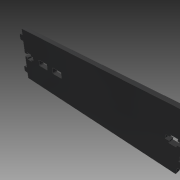
# Autodesk Inventor part: front_panel_2004_front
Saved by Autodesk Inventor 2014 (Build 180170000, 170)
## iProperties
Created: 2014-01-11
Part Number: front_panel_2004_front
Material: Generic
Document SubType Name: Modeling
Designer: buben
Density: 1 g/cm^3
Appearance: Anodized - Dark Gray
Author: buben
Autodesk Inventor part; units mm, degrees
ref_plane "YZ Plane" through (0, 0, 0) normal (1, 0, 0) x (0, 1, 0)
ref_plane "XZ Plane" through (0, 0, 0) normal (0, 1, 0) x (-1, 0, 0)
ref_plane "XY Plane" through (0, 0, 0) normal (0, 0, 1) x (1, 0, 0)
sketch "Sketch1" plane through (0, 0, 0) normal (0, 1, 0) x (-1, 0, 0)
  line L0 (0, 0) -> (220, 0)
  line L1 (220, 0) -> (220, 68.618)
  line L2 (220, 68.618) -> (0, 68.618)
  line L3 (0, 68.618) -> (0, 0)
  dimension "d0" = 68.618
  dimension "d1" = 220
  constraints: 8 end point, 2 parallel, 1 horizontal, 1 perpendicular
  measures "d0" distance of L2.end L0.start
  measures "d1" distance of L1.end L2.end
extrude "Extrusion1" add sketch "Sketch1" along normal blind 6
sketch "Sketch2" plane through (0, 6, 0) normal (0, 1, 0) x (1, 0, 0)
  line L0 (-220, 0) -> (-220, -68.618) projected
  line L1 (0, -68.618) -> (0, 0) projected
  line L2 (-220, -8) -> (-224, -8)
  line L3 (-226, -10) -> (-226, -14)
  line L4 (-224, -16) -> (-220, -16)
  line L5 (-220, -16) -> (-220, -8)
  line L6 (-220, -52.618) -> (-224, -52.618)
  line L7 (-226, -54.618) -> (-226, -58.618)
  line L8 (-224, -60.618) -> (-220, -60.618)
  line L9 (-220, -60.618) -> (-220, -52.618)
  line L10 (0, -8) -> (4, -8)
  line L11 (6, -10) -> (6, -14)
  line L12 (4, -16) -> (0, -16)
  line L13 (0, -16) -> (0, -8)
  line L14 (0, -52.618) -> (4, -52.618)
  line L15 (6, -54.618) -> (6, -58.618)
  line L16 (4, -60.618) -> (0, -60.618)
  line L17 (0, -60.618) -> (0, -52.618)
  arc A0 (-224, -8) -> (-226, -10) centre (-224, -10) ccw
  arc A1 (-226, -14) -> (-224, -16) centre (-224, -14) ccw
  arc A2 (-224, -52.618) -> (-226, -54.618) centre (-224, -54.618) ccw
  arc A3 (-226, -58.618) -> (-224, -60.618) centre (-224, -58.618) ccw
  arc A4 (4, -60.618) -> (6, -58.618) centre (4, -58.618) ccw
  arc A5 (6, -54.618) -> (4, -52.618) centre (4, -54.618) ccw
  arc A6 (4, -16) -> (6, -14) centre (4, -14) ccw
  arc A7 (6, -10) -> (4, -8) centre (4, -10) ccw
  line L18 (-222, -16) -> (-222, -52.618) construction
  line L19 (0, 0) -> (-220, 0) projected
  point P0 (-222, -34.309)
  point P1 (-220, -34.309)
  dimension "d4" = 2
  dimension "d5" = 8
  dimension "d6" = 8
  dimension "d7" = 6
  dimension "d8" = 6
  dimension "d41" = 8
  constraints: 34 end point, 16 point on circle, 16 tangent, 8 centre point, 8 parallel, 7 equal radius, 6 collinear, 4 horizontal, 4 midpoint, 4 perpendicular, 4 point on line, 1 horizontal alignment
  measures "d4" radius of A0
  measures "d5" distance between parallel lines of L4 L2
  measures "d6" distance between parallel lines of L8 L6
  measures "d7" distance between parallel lines of L0 L3
  measures "d8" distance between parallel lines of L1 L11
  measures "d41" distance between parallel lines of L19 L2
extrude "Extrusion2" add sketch "Sketch2" against normal blind 6
sketch "Sketch3" plane through (0, 6, 0) normal (0, 1, 0) x (1, 0, 0)
  line L0 (0, 0) -> (-220, 0) projected
  line L1 (-220, -16) -> (-220, -52.618) projected
  line L2 (-220, -68.618) -> (0, -68.618) projected
  line L3 (-203.7, -32.059) -> (-203.7, -36.559)
  line L4 (-220, -36.559) -> (-220, -32.059)
  line L5 (-215, -29.559) -> (-207.7, -29.559)
  line L6 (-207.7, -39.059) -> (-215, -39.059)
  line L7 (-220, -32.059) -> (-215, -32.059)
  line L8 (-207.7, -32.059) -> (-203.7, -32.059)
  line L9 (-203.7, -36.559) -> (-207.7, -36.559)
  line L10 (-215, -36.559) -> (-220, -36.559)
  line L11 (-207.7, -29.559) -> (-207.7, -32.059)
  line L12 (-207.7, -36.559) -> (-207.7, -39.059)
  line L13 (-215, -39.059) -> (-215, -36.559)
  line L14 (-215, -32.059) -> (-215, -29.559)
  line L15 (-110, 0) -> (-110, -68.618) construction
  line L16 (-16.3, -32.059) -> (-16.3, -36.559)
  line L17 (0, -36.559) -> (0, -32.059)
  line L18 (-5, -29.559) -> (-12.3, -29.559)
  line L19 (-12.3, -39.059) -> (-5, -39.059)
  line L20 (0, -32.059) -> (-5, -32.059)
  line L21 (-12.3, -32.059) -> (-16.3, -32.059)
  line L22 (-16.3, -36.559) -> (-12.3, -36.559)
  line L23 (-5, -36.559) -> (0, -36.559)
  line L24 (-12.3, -29.559) -> (-12.3, -32.059)
  line L25 (-12.3, -36.559) -> (-12.3, -39.059)
  line L26 (-5, -39.059) -> (-5, -36.559)
  line L27 (-5, -32.059) -> (-5, -29.559)
  point P0 (-203.7, -34.309)
  point P1 (-220, -34.309)
  point P2 (-16.3, -34.309)
  point P3 (0, -34.309)
  dimension "d12" = 4.5
  dimension "d13" = 2.5
  dimension "d14" = 2.5
  dimension "d15" = 5
  dimension "d16" = 4
  dimension "d17" = 7.3
  constraints: 50 end point, 14 symmetric about line, 10 parallel, 5 collinear, 4 midpoint, 4 perpendicular, 3 horizontal, 1 horizontal alignment
  measures "d12" distance of L3.start L3.end
  measures "d13" distance of L5.end L8.start
  measures "d14" distance of L9.end L6.start
  measures "d15" distance of L10.start L4.start
  measures "d16" distance of L3.end L9.end
  measures "d17" distance of L6.start L6.end
extrude "Extrusion3" cut sketch "Sketch3" against normal blind 6
sketch "Sketch4" plane through (0, 0, 0) normal (0, -1, 0) x (1, 0, 0)
  line L0 (-203.7, 36.559) -> (-203.7, 32.059) projected
  line L1 (-190.7, 38.309) -> (-177.7, 38.309)
  line L2 (-176.7, 37.309) -> (-176.7, 31.309)
  line L3 (-177.7, 30.309) -> (-190.7, 30.309)
  line L4 (-191.7, 31.309) -> (-191.7, 37.309)
  line L5 (-165.7, 38.309) -> (-152.7, 38.309)
  line L6 (-151.7, 37.309) -> (-151.7, 31.309)
  line L7 (-152.7, 30.309) -> (-165.7, 30.309)
  line L8 (-166.7, 31.309) -> (-166.7, 37.309)
  arc A0 (-190.7, 38.309) -> (-191.7, 37.309) centre (-190.7, 37.309) ccw
  arc A1 (-176.7, 37.309) -> (-177.7, 38.309) centre (-177.7, 37.309) ccw
  arc A2 (-177.7, 30.309) -> (-176.7, 31.309) centre (-177.7, 31.309) ccw
  arc A3 (-191.7, 31.309) -> (-190.7, 30.309) centre (-190.7, 31.309) ccw
  arc A4 (-165.7, 38.309) -> (-166.7, 37.309) centre (-165.7, 37.309) ccw
  arc A5 (-151.7, 37.309) -> (-152.7, 38.309) centre (-152.7, 37.309) ccw
  arc A6 (-152.7, 30.309) -> (-151.7, 31.309) centre (-152.7, 31.309) ccw
  arc A7 (-166.7, 31.309) -> (-165.7, 30.309) centre (-165.7, 31.309) ccw
  point P0 (-203.7, 34.309)
  point P1 (-191.7, 34.309)
  dimension "d20" = 1
  dimension "d21" = 15
  dimension "d22" = 15
  dimension "d23" = 8
  dimension "d24" = 10
  dimension "d25" = 12
  constraints: 16 end point, 16 point on circle, 16 tangent, 8 centre point, 7 equal radius, 4 parallel, 2 collinear, 2 horizontal, 2 midpoint, 2 perpendicular, 1 horizontal alignment
  measures "d20" radius of A0
  measures "d21" distance between parallel lines of L2 L4
  measures "d22" distance between parallel lines of L6 L8
  measures "d23" distance between parallel lines of L3 L1
  measures "d24" distance between parallel lines of L8 L2
  measures "d25" distance between parallel lines of L0 L4
extrude "Extrusion4" cut sketch "Sketch4" against normal through all
sketch "Sketch6" plane through (0, 6, 0) normal (0, 1, 0) x (1, 0, 0)
  line L0 (-220, -68.618) -> (0, -68.618) projected
  line L1 (0, -68.618) -> (0, -60.618) projected
  line L2 (-50, -52.618) -> (-10, -52.618) construction
  line L3 (-10, -52.618) -> (-10, -62.618) construction
  line L4 (-10, -62.618) -> (-50, -62.618) construction
  line L5 (-50, -62.618) -> (-50, -52.618) construction
  spline S0 degree 2 poles (-43.1283, -54.9198) (-43.1283, -55.8013) (-43.8661, -56.3008) knots 0 0 0 1 1 1
  spline S1 degree 2 poles (-43.8661, -56.3008) (-44.16, -56.4967) (-44.5518, -56.4967) knots 0 0 0 1 1 1
  line L6 (-44.5518, -56.4967) -> (-45.9035, -56.4967)
  spline S2 degree 2 poles (-45.9035, -56.4967) (-46.07, -56.4967) (-46.07, -56.3694) knots 0 0 0 1 1 1
  spline S3 degree 2 poles (-46.07, -56.3694) (-46.07, -56.2453) (-45.9035, -56.2453) knots 0 0 0 1 1 1
  line L7 (-45.9035, -56.2453) -> (-45.6912, -56.2453)
  line L8 (-45.6912, -56.2453) -> (-45.6912, -53.2481)
  line L9 (-45.6912, -53.2481) -> (-45.9035, -53.2481)
  spline S4 degree 2 poles (-45.9035, -53.2481) (-46.07, -53.2481) (-46.07, -53.1208) knots 0 0 0 1 1 1
  spline S5 degree 2 poles (-46.07, -53.1208) (-46.07, -52.9967) (-45.9035, -52.9967) knots 0 0 0 1 1 1
  line L10 (-45.9035, -52.9967) -> (-44.5518, -52.9967)
  spline S6 degree 2 poles (-44.5518, -52.9967) (-43.9282, -52.9967) (-43.5723, -53.4277) knots 0 0 0 1 1 1
  spline S7 degree 2 poles (-43.5723, -53.4277) (-43.1283, -53.9664) (-43.1283, -54.5737) knots 0 0 0 1 1 1
  line L11 (-43.1283, -54.5737) -> (-43.1283, -54.9198)
  line L12 (-43.3797, -54.9753) -> (-43.3797, -54.5182)
  spline S8 degree 2 poles (-43.3797, -54.5182) (-43.3797, -54.2864) (-43.4548, -54.1035) knots 0 0 0 1 1 1
  spline S9 degree 2 poles (-43.4548, -54.1035) (-43.5625, -53.8358) (-43.7584, -53.5975) knots 0 0 0 1 1 1
  spline S10 degree 2 poles (-43.7584, -53.5975) (-44.0457, -53.2481) (-44.5289, -53.2481) knots 0 0 0 1 1 1
  line L13 (-44.5289, -53.2481) -> (-45.4398, -53.2481)
  line L14 (-45.4398, -53.2481) -> (-45.4398, -56.2453)
  line L15 (-45.4398, -56.2453) -> (-44.5289, -56.2453)
  spline S11 degree 2 poles (-44.5289, -56.2453) (-44.2155, -56.2453) (-43.9314, -56.0364) knots 0 0 0 1 1 1
  spline S12 degree 2 poles (-43.9314, -56.0364) (-43.6604, -55.8405) (-43.5168, -55.5434) knots 0 0 0 1 1 1
  spline S13 degree 2 poles (-43.5168, -55.5434) (-43.3797, -55.2561) (-43.3797, -54.9753) knots 0 0 0 1 1 1
  spline S14 degree 2 poles (-39.6642, -56.0854) (-39.6642, -56.1343) (-39.7132, -56.1866) knots 0 0 0 1 1 1
  spline S15 degree 2 poles (-39.7132, -56.1866) (-39.896, -56.3727) (-40.3041, -56.4935) knots 0 0 0 1 1 1
  spline S16 degree 2 poles (-40.3041, -56.4935) (-40.66, -56.5947) (-40.9734, -56.5947) knots 0 0 0 1 1 1
  spline S17 degree 2 poles (-40.9734, -56.5947) (-41.6035, -56.5947) (-42.0378, -56.1866) knots 0 0 0 1 1 1
  spline S18 degree 2 poles (-42.0378, -56.1866) (-42.4851, -55.7719) (-42.4851, -55.1483) knots 0 0 0 1 1 1
  spline S19 degree 2 poles (-42.4851, -55.1483) (-42.4851, -54.5737) (-42.0639, -54.1884) knots 0 0 0 1 1 1
  spline S20 degree 2 poles (-42.0639, -54.1884) (-41.6525, -53.8162) (-41.0779, -53.8162) knots 0 0 0 1 1 1
  spline S21 degree 2 poles (-41.0779, -53.8162) (-40.4445, -53.8162) (-39.6642, -54.6292) (-39.6707, -55.2626) knots 0 0 0 1 2 2 2
  line L16 (-39.6707, -55.2626) -> (-42.2304, -55.2626)
  spline S22 degree 2 poles (-42.2304, -55.2626) (-42.1651, -55.7589) (-41.4762, -56.3433) (-40.9734, -56.3433) knots 0 0 0 1 2 2 2
  spline S23 degree 2 poles (-40.9734, -56.3433) (-40.3139, -56.3433) (-39.8829, -56.007) knots 0 0 0 1 1 1
  spline S24 degree 2 poles (-39.8829, -56.007) (-39.8242, -55.9613) (-39.785, -55.9613) knots 0 0 0 1 1 1
  spline S25 degree 2 poles (-39.785, -55.9613) (-39.6642, -55.9613) (-39.6642, -56.0854) knots 0 0 0 1 1 1
  spline S26 degree 2 poles (-39.9254, -55.0079) (-40.0005, -54.5835) (-40.6437, -54.0709) (-41.0746, -54.0709) knots 0 0 0 1 2 2 2
  spline S27 degree 2 poles (-41.0746, -54.0709) (-41.5121, -54.0709) (-42.1488, -54.5802) (-42.2271, -55.0079) knots 0 0 0 1 2 2 2
  line L17 (-42.2271, -55.0079) -> (-39.9254, -55.0079)
  spline S28 degree 2 poles (-36.1348, -55.7752) (-36.1348, -56.1931) (-36.5527, -56.4151) knots 0 0 0 1 1 1
  spline S29 degree 2 poles (-36.5527, -56.4151) (-36.8923, -56.5947) (-37.3461, -56.5947) knots 0 0 0 1 1 1
  spline S30 degree 2 poles (-37.3461, -56.5947) (-37.9403, -56.5947) (-38.319, -56.2943) knots 0 0 0 1 1 1
  spline S31 degree 2 poles (-38.319, -56.2943) (-38.319, -56.4412) (-38.3713, -56.4771) knots 0 0 0 1 1 1
  spline S32 degree 2 poles (-38.3713, -56.4771) (-38.4072, -56.4967) (-38.4431, -56.4967) knots 0 0 0 1 1 1
  spline S33 degree 2 poles (-38.4431, -56.4967) (-38.5704, -56.4967) (-38.5704, -56.3302) knots 0 0 0 1 1 1
  line L18 (-38.5704, -56.3302) -> (-38.5704, -55.8111)
  spline S34 degree 2 poles (-38.5704, -55.8111) (-38.5704, -55.6446) (-38.4431, -55.6446) knots 0 0 0 1 1 1
  spline S35 degree 2 poles (-38.4431, -55.6446) (-38.3158, -55.6446) (-38.3158, -55.7817) knots 0 0 0 1 1 1
  spline S36 degree 2 poles (-38.3158, -55.7817) (-38.3158, -56.0821) (-37.9109, -56.2486) knots 0 0 0 1 1 1
  spline S37 degree 2 poles (-37.9109, -56.2486) (-37.6856, -56.3433) (-37.3526, -56.3433) knots 0 0 0 1 1 1
  spline S38 degree 2 poles (-37.3526, -56.3433) (-37.0163, -56.3433) (-36.7486, -56.2257) knots 0 0 0 1 1 1
  spline S39 degree 2 poles (-36.7486, -56.2257) (-36.3862, -56.0723) (-36.3862, -55.7752) knots 0 0 0 1 1 1
  spline S40 degree 2 poles (-36.3862, -55.7752) (-36.3862, -55.3116) (-37.3396, -55.2136) knots 0 0 0 1 1 1
  spline S41 degree 2 poles (-37.3396, -55.2136) (-37.715, -55.1744) (-37.8783, -55.1287) knots 0 0 0 1 1 1
  spline S42 degree 2 poles (-37.8783, -55.1287) (-38.1884, -55.0438) (-38.3288, -54.8545) knots 0 0 0 1 1 1
  spline S43 degree 2 poles (-38.3288, -54.8545) (-38.4431, -54.6978) (-38.4431, -54.5182) knots 0 0 0 1 1 1
  spline S44 degree 2 poles (-38.4431, -54.5182) (-38.4431, -54.1623) (-38.0644, -53.9697) knots 0 0 0 1 1 1
  spline S45 degree 2 poles (-38.0644, -53.9697) (-37.7607, -53.8162) (-37.3689, -53.8162) knots 0 0 0 1 1 1
  spline S46 degree 2 poles (-37.3689, -53.8162) (-36.8498, -53.8162) (-36.5233, -54.0676) knots 0 0 0 1 1 1
  spline S47 degree 2 poles (-36.5233, -54.0676) (-36.5233, -53.9044) (-36.396, -53.9044) knots 0 0 0 1 1 1
  spline S48 degree 2 poles (-36.396, -53.9044) (-36.2687, -53.9044) (-36.2687, -54.0742) knots 0 0 0 1 1 1
  line L19 (-36.2687, -54.0742) -> (-36.2687, -54.5084)
  spline S49 degree 2 poles (-36.2687, -54.5084) (-36.2687, -54.6749) (-36.396, -54.6749) knots 0 0 0 1 1 1
  spline S50 degree 2 poles (-36.396, -54.6749) (-36.5103, -54.6749) (-36.5233, -54.5345) knots 0 0 0 1 1 1
  spline S51 degree 2 poles (-36.5233, -54.5345) (-36.5396, -54.3549) (-36.7094, -54.2374) knots 0 0 0 1 1 1
  spline S52 degree 2 poles (-36.7094, -54.2374) (-36.951, -54.0709) (-37.3559, -54.0709) knots 0 0 0 1 1 1
  spline S53 degree 2 poles (-37.3559, -54.0709) (-37.7803, -54.0709) (-38.0121, -54.2407) knots 0 0 0 1 1 1
  spline S54 degree 2 poles (-38.0121, -54.2407) (-38.1884, -54.3713) (-38.1884, -54.528) knots 0 0 0 1 1 1
  spline S55 degree 2 poles (-38.1884, -54.528) (-38.1884, -54.7076) (-37.9795, -54.8284) knots 0 0 0 1 1 1
  spline S56 degree 2 poles (-37.9795, -54.8284) (-37.8326, -54.91) (-37.4342, -54.9557) knots 0 0 0 1 1 1
  spline S57 degree 2 poles (-37.4342, -54.9557) (-36.9053, -55.0145) (-36.7094, -55.083) knots 0 0 0 1 1 1
  spline S58 degree 2 poles (-36.7094, -55.083) (-36.1348, -55.292) (-36.1348, -55.7752) knots 0 0 0 1 1 1
  spline S59 degree 2 poles (-32.3867, -56.3694) (-32.3867, -56.4967) (-32.5564, -56.4967) knots 0 0 0 1 1 1
  line L20 (-32.5564, -56.4967) -> (-34.7831, -56.4967)
  spline S60 degree 2 poles (-34.7831, -56.4967) (-34.9496, -56.4967) (-34.9496, -56.3694) knots 0 0 0 1 1 1
  spline S61 degree 2 poles (-34.9496, -56.3694) (-34.9496, -56.2453) (-34.7831, -56.2453) knots 0 0 0 1 1 1
  line L21 (-34.7831, -56.2453) -> (-33.7938, -56.2453)
  line L22 (-33.7938, -56.2453) -> (-33.7938, -54.1623)
  line L23 (-33.7938, -54.1623) -> (-34.5285, -54.1623)
  spline S62 degree 2 poles (-34.5285, -54.1623) (-34.6982, -54.1623) (-34.6982, -54.035) knots 0 0 0 1 1 1
  spline S63 degree 2 poles (-34.6982, -54.035) (-34.6982, -53.9076) (-34.5285, -53.9076) knots 0 0 0 1 1 1
  line L24 (-34.5285, -53.9076) -> (-33.5424, -53.9076)
  line L25 (-33.5424, -53.9076) -> (-33.5424, -56.2453)
  line L26 (-33.5424, -56.2453) -> (-32.5564, -56.2453)
  spline S64 degree 2 poles (-32.5564, -56.2453) (-32.3867, -56.2453) (-32.3867, -56.3694) knots 0 0 0 1 1 1
  line L27 (-33.549, -53.2677) -> (-33.9212, -53.2677)
  line L28 (-33.9212, -53.2677) -> (-33.9212, -52.618)
  line L29 (-33.9212, -52.618) -> (-33.549, -52.618)
  line L30 (-33.549, -52.618) -> (-33.549, -53.2677)
  spline S65 degree 2 poles (-28.3969, -54.035) (-28.3969, -54.1623) (-28.5634, -54.1623) knots 0 0 0 1 1 1
  line L31 (-28.5634, -54.1623) -> (-28.903, -54.1623)
  line L32 (-28.903, -54.1623) -> (-28.903, -56.6698)
  spline S66 degree 2 poles (-28.903, -56.6698) (-28.903, -56.9212) (-29.0107, -57.1171) knots 0 0 0 1 1 1
  spline S67 degree 2 poles (-29.0107, -57.1171) (-29.1772, -57.424) (-29.556, -57.5905) knots 0 0 0 1 1 1
  spline S68 degree 2 poles (-29.556, -57.5905) (-29.6931, -57.6493) (-29.9249, -57.6493) knots 0 0 0 1 1 1
  line L33 (-29.9249, -57.6493) -> (-30.6367, -57.6493)
  spline S69 degree 2 poles (-30.6367, -57.6493) (-30.8032, -57.6493) (-30.8032, -57.5219) knots 0 0 0 1 1 1
  spline S70 degree 2 poles (-30.8032, -57.5219) (-30.8032, -57.3946) (-30.6367, -57.3946) knots 0 0 0 1 1 1
  line L34 (-30.6367, -57.3946) -> (-29.9151, -57.3979)
  spline S71 degree 2 poles (-29.9151, -57.3979) (-29.458, -57.4011) (-29.2197, -56.9538) knots 0 0 0 1 1 1
  spline S72 degree 2 poles (-29.2197, -56.9538) (-29.1544, -56.8298) (-29.1544, -56.6339) knots 0 0 0 1 1 1
  line L35 (-29.1544, -56.6339) -> (-29.1544, -55.8797)
  spline S73 degree 2 poles (-29.1544, -55.8797) (-29.5592, -56.4347) (-30.1959, -56.4347) knots 0 0 0 1 1 1
  spline S74 degree 2 poles (-30.1959, -56.4347) (-30.7281, -56.4347) (-31.097, -56.0429) knots 0 0 0 1 1 1
  spline S75 degree 2 poles (-31.097, -56.0429) (-31.4627, -55.6609) (-31.4627, -55.1255) knots 0 0 0 1 1 1
  spline S76 degree 2 poles (-31.4627, -55.1255) (-31.4627, -54.5868) (-30.7281, -53.8162) (-30.1959, -53.8162) knots 0 0 0 1 2 2 2
  spline S77 degree 2 poles (-30.1959, -53.8162) (-29.5592, -53.8162) (-29.1544, -54.368) knots 0 0 0 1 1 1
  line L36 (-29.1544, -54.368) -> (-29.1544, -53.9076)
  line L37 (-29.1544, -53.9076) -> (-28.5634, -53.9076)
  spline S78 degree 2 poles (-28.5634, -53.9076) (-28.3969, -53.9076) (-28.3969, -54.035) knots 0 0 0 1 1 1
  spline S79 degree 2 poles (-29.1544, -55.1255) (-29.1544, -54.688) (-29.7486, -54.0709) (-30.1828, -54.0709) knots 0 0 0 1 2 2 2
  spline S80 degree 2 poles (-30.1828, -54.0709) (-30.6171, -54.0709) (-31.208, -54.6912) (-31.208, -55.1255) knots 0 0 0 1 2 2 2
  spline S81 degree 2 poles (-31.208, -55.1255) (-31.208, -55.5597) (-30.6171, -56.18) (-30.1828, -56.18) knots 0 0 0 1 2 2 2
  spline S82 degree 2 poles (-30.1828, -56.18) (-29.7486, -56.18) (-29.1544, -55.5597) (-29.1544, -55.1255) knots 0 0 0 1 2 2 2
  spline S83 degree 2 poles (-24.8414, -56.3694) (-24.8414, -56.4967) (-25.0079, -56.4967) knots 0 0 0 1 1 1
  line L38 (-25.0079, -56.4967) -> (-25.6805, -56.4967)
  spline S84 degree 2 poles (-25.6805, -56.4967) (-25.8503, -56.4967) (-25.8503, -56.3694) knots 0 0 0 1 1 1
  spline S85 degree 2 poles (-25.8503, -56.3694) (-25.8503, -56.2453) (-25.6805, -56.2453) knots 0 0 0 1 1 1
  line L39 (-25.6805, -56.2453) -> (-25.4715, -56.2453)
  line L40 (-25.4715, -56.2453) -> (-25.4715, -54.7043)
  spline S86 degree 2 poles (-25.4715, -54.7043) (-25.4715, -54.4104) (-25.687, -54.2341) knots 0 0 0 1 1 1
  spline S87 degree 2 poles (-25.687, -54.2341) (-25.8862, -54.0709) (-26.1866, -54.0709) knots 0 0 0 1 1 1
  spline S88 degree 2 poles (-26.1866, -54.0709) (-26.4902, -54.0709) (-26.7285, -54.2472) knots 0 0 0 1 1 1
  spline S89 degree 2 poles (-26.7285, -54.2472) (-26.8657, -54.3484) (-27.1367, -54.6684) knots 0 0 0 1 1 1
  line L41 (-27.1367, -54.6684) -> (-27.1367, -56.2453)
  line L42 (-27.1367, -56.2453) -> (-26.8526, -56.2453)
  spline S90 degree 2 poles (-26.8526, -56.2453) (-26.6861, -56.2453) (-26.6861, -56.3694) knots 0 0 0 1 1 1
  spline S91 degree 2 poles (-26.6861, -56.3694) (-26.6861, -56.4967) (-26.8526, -56.4967) knots 0 0 0 1 1 1
  line L43 (-26.8526, -56.4967) -> (-27.6721, -56.4967)
  spline S92 degree 2 poles (-27.6721, -56.4967) (-27.8386, -56.4967) (-27.8386, -56.3694) knots 0 0 0 1 1 1
  spline S93 degree 2 poles (-27.8386, -56.3694) (-27.8386, -56.2453) (-27.6721, -56.2453) knots 0 0 0 1 1 1
  line L44 (-27.6721, -56.2453) -> (-27.3881, -56.2453)
  line L45 (-27.3881, -56.2453) -> (-27.3881, -54.1623)
  line L46 (-27.3881, -54.1623) -> (-27.6003, -54.1623)
  spline S94 degree 2 poles (-27.6003, -54.1623) (-27.7668, -54.1623) (-27.7668, -54.035) knots 0 0 0 1 1 1
  spline S95 degree 2 poles (-27.7668, -54.035) (-27.7668, -53.9076) (-27.6003, -53.9076) knots 0 0 0 1 1 1
  line L47 (-27.6003, -53.9076) -> (-27.1367, -53.9076)
  line L48 (-27.1367, -53.9076) -> (-27.1367, -54.2864)
  spline S96 degree 2 poles (-27.1367, -54.2864) (-26.673, -53.8162) (-26.1833, -53.8162) knots 0 0 0 1 1 1
  spline S97 degree 2 poles (-26.1833, -53.8162) (-25.6283, -53.8162) (-25.354, -54.2341) knots 0 0 0 1 1 1
  spline S98 degree 2 poles (-25.354, -54.2341) (-25.2201, -54.4431) (-25.2201, -54.6618) knots 0 0 0 1 1 1
  line L49 (-25.2201, -54.6618) -> (-25.2201, -56.2453)
  line L50 (-25.2201, -56.2453) -> (-25.0079, -56.2453)
  spline S99 degree 2 poles (-25.0079, -56.2453) (-24.8414, -56.2453) (-24.8414, -56.3694) knots 0 0 0 1 1 1
  spline S100 degree 2 poles (-17.4855, -55.194) (-17.4855, -55.7621) (-17.8643, -56.1735) knots 0 0 0 1 1 1
  spline S101 degree 2 poles (-17.8643, -56.1735) (-18.2528, -56.5947) (-18.8209, -56.5947) knots 0 0 0 1 1 1
  spline S102 degree 2 poles (-18.8209, -56.5947) (-19.4771, -56.5947) (-19.9179, -56.0037) knots 0 0 0 1 1 1
  line L51 (-19.9179, -56.0037) -> (-19.9179, -56.4967)
  line L52 (-19.9179, -56.4967) -> (-20.5089, -56.4967)
  spline S103 degree 2 poles (-20.5089, -56.4967) (-20.6754, -56.4967) (-20.6754, -56.3694) knots 0 0 0 1 1 1
  spline S104 degree 2 poles (-20.6754, -56.3694) (-20.6754, -56.2453) (-20.5089, -56.2453) knots 0 0 0 1 1 1
  line L53 (-20.5089, -56.2453) -> (-20.1693, -56.2453)
  line L54 (-20.1693, -56.2453) -> (-20.1693, -52.9967)
  line L55 (-20.1693, -52.9967) -> (-20.5089, -52.9967)
  spline S105 degree 2 poles (-20.5089, -52.9967) (-20.6754, -52.9967) (-20.6754, -52.8694) knots 0 0 0 1 1 1
  spline S106 degree 2 poles (-20.6754, -52.8694) (-20.6754, -52.7421) (-20.5089, -52.7421) knots 0 0 0 1 1 1
  line L56 (-20.5089, -52.7421) -> (-19.9179, -52.7421)
  line L57 (-19.9179, -52.7421) -> (-19.9179, -54.4072)
  spline S107 degree 2 poles (-19.9179, -54.4072) (-19.4641, -53.8162) (-18.8209, -53.8162) knots 0 0 0 1 1 1
  spline S108 degree 2 poles (-18.8209, -53.8162) (-18.2528, -53.8162) (-17.4855, -54.6227) (-17.4855, -55.194) knots 0 0 0 1 2 2 2
  spline S109 degree 2 poles (-17.7369, -55.2071) (-17.7369, -54.7467) (-18.0471, -54.4104) knots 0 0 0 1 1 1
  spline S110 degree 2 poles (-18.0471, -54.4104) (-18.3671, -54.0709) (-18.8242, -54.0709) knots 0 0 0 1 1 1
  spline S111 degree 2 poles (-18.8242, -54.0709) (-19.2845, -54.0709) (-19.9146, -54.7467) (-19.9146, -55.2071) knots 0 0 0 1 2 2 2
  spline S112 degree 2 poles (-19.9146, -55.2071) (-19.9146, -55.6674) (-19.2845, -56.3433) (-18.8242, -56.3433) knots 0 0 0 1 2 2 2
  spline S113 degree 2 poles (-18.8242, -56.3433) (-18.3671, -56.3433) (-18.0471, -56.0037) knots 0 0 0 1 1 1
  spline S114 degree 2 poles (-18.0471, -56.0037) (-17.7369, -55.6674) (-17.7369, -55.2071) knots 0 0 0 1 1 1
  spline S115 degree 2 poles (-13.6199, -54.035) (-13.6199, -54.1231) (-13.6982, -54.1493) knots 0 0 0 1 1 1
  spline S116 degree 2 poles (-13.6982, -54.1493) (-13.7276, -54.1623) (-13.8647, -54.1623) knots 0 0 0 1 1 1
  line L58 (-13.8647, -54.1623) -> (-15.4515, -57.3979)
  line L59 (-15.4515, -57.3979) -> (-15.0597, -57.3979)
  spline S117 degree 2 poles (-15.0597, -57.3979) (-14.8932, -57.3979) (-14.8932, -57.5219) knots 0 0 0 1 1 1
  spline S118 degree 2 poles (-14.8932, -57.5219) (-14.8932, -57.6493) (-15.0597, -57.6493) knots 0 0 0 1 1 1
  line L60 (-15.0597, -57.6493) -> (-16.5093, -57.6493)
  spline S119 degree 2 poles (-16.5093, -57.6493) (-16.6758, -57.6493) (-16.6758, -57.5219) knots 0 0 0 1 1 1
  spline S120 degree 2 poles (-16.6758, -57.5219) (-16.6758, -57.3979) (-16.5093, -57.3979) knots 0 0 0 1 1 1
  line L61 (-16.5093, -57.3979) -> (-15.7225, -57.3979)
  line L62 (-15.7225, -57.3979) -> (-15.2785, -56.4967)
  line L63 (-15.2785, -56.4967) -> (-16.4473, -54.1623)
  line L64 (-16.4473, -54.1623) -> (-16.5224, -54.1623)
  spline S121 degree 2 poles (-16.5224, -54.1623) (-16.6889, -54.1623) (-16.6889, -54.035) knots 0 0 0 1 1 1
  spline S122 degree 2 poles (-16.6889, -54.035) (-16.6889, -53.9534) (-16.6171, -53.9207) knots 0 0 0 1 1 1
  spline S123 degree 2 poles (-16.6171, -53.9207) (-16.5877, -53.9076) (-16.5224, -53.9076) knots 0 0 0 1 1 1
  line L65 (-16.5224, -53.9076) -> (-15.8335, -53.9076)
  spline S124 degree 2 poles (-15.8335, -53.9076) (-15.667, -53.9076) (-15.667, -54.035) knots 0 0 0 1 1 1
  spline S125 degree 2 poles (-15.667, -54.035) (-15.667, -54.1623) (-15.8335, -54.1623) knots 0 0 0 1 1 1
  line L66 (-15.8335, -54.1623) -> (-16.173, -54.1623)
  line L67 (-16.173, -54.1623) -> (-15.1413, -56.2192)
  line L68 (-15.1413, -56.2192) -> (-14.1357, -54.1623)
  line L69 (-14.1357, -54.1623) -> (-14.4753, -54.1623)
  spline S126 degree 2 poles (-14.4753, -54.1623) (-14.6418, -54.1623) (-14.6418, -54.035) knots 0 0 0 1 1 1
  spline S127 degree 2 poles (-14.6418, -54.035) (-14.6418, -53.9076) (-14.4753, -53.9076) knots 0 0 0 1 1 1
  line L70 (-14.4753, -53.9076) -> (-13.7896, -53.9076)
  spline S128 degree 2 poles (-13.7896, -53.9076) (-13.6199, -53.9076) (-13.6199, -54.035) knots 0 0 0 1 1 1
  spline S129 degree 2 poles (-47.2257, -62.1623) (-47.2257, -62.2897) (-47.3923, -62.2897) knots 0 0 0 1 1 1
  line L71 (-47.3923, -62.2897) -> (-49.3675, -62.2897)
  spline S130 degree 2 poles (-49.3675, -62.2897) (-49.534, -62.2897) (-49.534, -62.1623) knots 0 0 0 1 1 1
  spline S131 degree 2 poles (-49.534, -62.1623) (-49.534, -62.0383) (-49.3675, -62.0383) knots 0 0 0 1 1 1
  line L72 (-49.3675, -62.0383) -> (-48.5056, -62.0383)
  line L73 (-48.5056, -62.0383) -> (-48.5056, -59.0411)
  line L74 (-48.5056, -59.0411) -> (-49.3675, -59.0411)
  spline S132 degree 2 poles (-49.3675, -59.0411) (-49.534, -59.0411) (-49.534, -58.9137) knots 0 0 0 1 1 1
  spline S133 degree 2 poles (-49.534, -58.9137) (-49.534, -58.7897) (-49.3675, -58.7897) knots 0 0 0 1 1 1
  line L75 (-49.3675, -58.7897) -> (-47.3923, -58.7897)
  spline S134 degree 2 poles (-47.3923, -58.7897) (-47.2257, -58.7897) (-47.2257, -58.9137) knots 0 0 0 1 1 1
  spline S135 degree 2 poles (-47.2257, -58.9137) (-47.2257, -59.0411) (-47.3923, -59.0411) knots 0 0 0 1 1 1
  line L76 (-47.3923, -59.0411) -> (-48.2542, -59.0411)
  line L77 (-48.2542, -59.0411) -> (-48.2542, -62.0383)
  line L78 (-48.2542, -62.0383) -> (-47.3923, -62.0383)
  spline S136 degree 2 poles (-47.3923, -62.0383) (-47.2257, -62.0383) (-47.2257, -62.1623) knots 0 0 0 1 1 1
  spline S137 degree 2 poles (-43.0466, -59.8279) (-43.0466, -59.9552) (-43.2132, -59.9552) knots 0 0 0 1 1 1
  line L79 (-43.2132, -59.9552) -> (-43.4678, -59.9552)
  line L80 (-43.4678, -59.9552) -> (-44.4865, -62.2897)
  line L81 (-44.4865, -62.2897) -> (-44.9109, -62.2897)
  line L82 (-44.9109, -62.2897) -> (-45.9426, -59.9552)
  line L83 (-45.9426, -59.9552) -> (-46.2006, -59.9552)
  spline S138 degree 2 poles (-46.2006, -59.9552) (-46.3671, -59.9552) (-46.3671, -59.8279) knots 0 0 0 1 1 1
  spline S139 degree 2 poles (-46.3671, -59.8279) (-46.3671, -59.7006) (-46.2006, -59.7006) knots 0 0 0 1 1 1
  line L84 (-46.2006, -59.7006) -> (-45.257, -59.7006)
  spline S140 degree 2 poles (-45.257, -59.7006) (-45.0905, -59.7006) (-45.0905, -59.8279) knots 0 0 0 1 1 1
  spline S141 degree 2 poles (-45.0905, -59.8279) (-45.0905, -59.9552) (-45.257, -59.9552) knots 0 0 0 1 1 1
  line L85 (-45.257, -59.9552) -> (-45.6716, -59.9552)
  line L86 (-45.6716, -59.9552) -> (-44.7509, -62.0383)
  line L87 (-44.7509, -62.0383) -> (-44.6465, -62.0383)
  line L88 (-44.6465, -62.0383) -> (-43.7388, -59.9552)
  line L89 (-43.7388, -59.9552) -> (-44.16, -59.9552)
  spline S142 degree 2 poles (-44.16, -59.9552) (-44.3265, -59.9552) (-44.3265, -59.8279) knots 0 0 0 1 1 1
  spline S143 degree 2 poles (-44.3265, -59.8279) (-44.3265, -59.7006) (-44.16, -59.7006) knots 0 0 0 1 1 1
  line L90 (-44.16, -59.7006) -> (-43.2132, -59.7006)
  spline S144 degree 2 poles (-43.2132, -59.7006) (-43.0466, -59.7006) (-43.0466, -59.8279) knots 0 0 0 1 1 1
  spline S145 degree 2 poles (-39.625, -61) (-39.625, -61.5812) (-40.4445, -62.3876) (-41.0289, -62.3876) knots 0 0 0 1 2 2 2
  spline S146 degree 2 poles (-41.0289, -62.3876) (-41.6101, -62.3876) (-42.4328, -61.5844) (-42.4328, -61) knots 0 0 0 1 2 2 2
  spline S147 degree 2 poles (-42.4328, -61) (-42.4328, -60.4156) (-41.6101, -59.6091) (-41.0289, -59.6091) knots 0 0 0 1 2 2 2
  spline S148 degree 2 poles (-41.0289, -59.6091) (-40.4445, -59.6091) (-39.625, -60.4156) (-39.625, -61) knots 0 0 0 1 2 2 2
  spline S149 degree 2 poles (-39.8797, -61) (-39.8797, -60.5201) (-40.5522, -59.8638) (-41.0289, -59.8638) knots 0 0 0 1 2 2 2
  spline S150 degree 2 poles (-41.0289, -59.8638) (-41.5089, -59.8638) (-42.1814, -60.5233) (-42.1814, -61) knots 0 0 0 1 2 2 2
  spline S151 degree 2 poles (-42.1814, -61) (-42.1814, -61.4767) (-41.5056, -62.1362) (-41.0289, -62.1362) knots 0 0 0 1 2 2 2
  spline S152 degree 2 poles (-41.0289, -62.1362) (-40.5522, -62.1362) (-39.8797, -61.4767) (-39.8797, -61) knots 0 0 0 1 2 2 2
  spline S153 degree 2 poles (-32.3899, -61.3494) (-32.3899, -61.8424) (-32.7915, -62.1297) knots 0 0 0 1 1 1
  spline S154 degree 2 poles (-32.7915, -62.1297) (-33.1507, -62.3876) (-33.6632, -62.3876) knots 0 0 0 1 1 1
  spline S155 degree 2 poles (-33.6632, -62.3876) (-34.3195, -62.3876) (-34.7113, -61.9795) knots 0 0 0 1 1 1
  line L91 (-34.7113, -61.9795) -> (-34.7113, -62.1231)
  spline S156 degree 2 poles (-34.7113, -62.1231) (-34.7113, -62.2897) (-34.8354, -62.2897) knots 0 0 0 1 1 1
  spline S157 degree 2 poles (-34.8354, -62.2897) (-34.9627, -62.2897) (-34.9627, -62.1231) knots 0 0 0 1 1 1
  line L92 (-34.9627, -62.1231) -> (-34.9627, -61.4277)
  spline S158 degree 2 poles (-34.9627, -61.4277) (-34.9627, -61.2579) (-34.8354, -61.2579) knots 0 0 0 1 1 1
  spline S159 degree 2 poles (-34.8354, -61.2579) (-34.7211, -61.2579) (-34.7113, -61.4114) knots 0 0 0 1 1 1
  spline S160 degree 2 poles (-34.7113, -61.4114) (-34.6917, -61.7607) (-34.3358, -61.9632) knots 0 0 0 1 1 1
  spline S161 degree 2 poles (-34.3358, -61.9632) (-34.0387, -62.1362) (-33.6632, -62.1362) knots 0 0 0 1 1 1
  spline S162 degree 2 poles (-33.6632, -62.1362) (-33.2617, -62.1362) (-32.9743, -61.9436) knots 0 0 0 1 1 1
  spline S163 degree 2 poles (-32.9743, -61.9436) (-32.6413, -61.7248) (-32.6413, -61.3428) knots 0 0 0 1 1 1
  spline S164 degree 2 poles (-32.6413, -61.3428) (-32.6413, -60.9282) (-33.0592, -60.7453) knots 0 0 0 1 1 1
  spline S165 degree 2 poles (-33.0592, -60.7453) (-33.2062, -60.68) (-33.6567, -60.605) knots 0 0 0 1 1 1
  spline S166 degree 2 poles (-33.6567, -60.605) (-34.1954, -60.5168) (-34.4534, -60.3568) knots 0 0 0 1 1 1
  spline S167 degree 2 poles (-34.4534, -60.3568) (-34.8354, -60.1283) (-34.8354, -59.6712) knots 0 0 0 1 1 1
  spline S168 degree 2 poles (-34.8354, -59.6712) (-34.8354, -59.2272) (-34.4729, -58.9529) knots 0 0 0 1 1 1
  spline S169 degree 2 poles (-34.4729, -58.9529) (-34.1465, -58.708) (-33.6828, -58.708) knots 0 0 0 1 1 1
  spline S170 degree 2 poles (-33.6828, -58.708) (-33.1572, -58.708) (-32.7752, -59.0411) knots 0 0 0 1 1 1
  line L93 (-32.7752, -59.0411) -> (-32.7752, -58.9562)
  spline S171 degree 2 poles (-32.7752, -58.9562) (-32.7752, -58.7897) (-32.6479, -58.7897) knots 0 0 0 1 1 1
  spline S172 degree 2 poles (-32.6479, -58.7897) (-32.5238, -58.7897) (-32.5238, -58.9562) knots 0 0 0 1 1 1
  line L94 (-32.5238, -58.9562) -> (-32.5238, -59.5961)
  spline S173 degree 2 poles (-32.5238, -59.5961) (-32.5238, -59.7626) (-32.6479, -59.7626) knots 0 0 0 1 1 1
  spline S174 degree 2 poles (-32.6479, -59.7626) (-32.7654, -59.7626) (-32.7752, -59.6091) knots 0 0 0 1 1 1
  spline S175 degree 2 poles (-32.7752, -59.6091) (-32.7948, -59.3055) (-33.0886, -59.1194) knots 0 0 0 1 1 1
  spline S176 degree 2 poles (-33.0886, -59.1194) (-33.3498, -58.9594) (-33.6763, -58.9594) knots 0 0 0 1 1 1
  spline S177 degree 2 poles (-33.6763, -58.9594) (-34.0322, -58.9594) (-34.2901, -59.1357) knots 0 0 0 1 1 1
  spline S178 degree 2 poles (-34.2901, -59.1357) (-34.584, -59.3382) (-34.584, -59.6777) knots 0 0 0 1 1 1
  spline S179 degree 2 poles (-34.584, -59.6777) (-34.584, -59.9814) (-34.3326, -60.1479) knots 0 0 0 1 1 1
  spline S180 degree 2 poles (-34.3326, -60.1479) (-34.1269, -60.285) (-33.6241, -60.3699) knots 0 0 0 1 1 1
  spline S181 degree 2 poles (-33.6241, -60.3699) (-33.1082, -60.4548) (-32.9188, -60.5397) knots 0 0 0 1 1 1
  spline S182 degree 2 poles (-32.9188, -60.5397) (-32.3899, -60.778) (-32.3899, -61.3494) knots 0 0 0 1 1 1
  spline S183 degree 2 poles (-28.7169, -62.1623) (-28.7169, -62.2897) (-28.8867, -62.2897) knots 0 0 0 1 1 1
  line L95 (-28.8867, -62.2897) -> (-31.1133, -62.2897)
  spline S184 degree 2 poles (-31.1133, -62.2897) (-31.2799, -62.2897) (-31.2799, -62.1623) knots 0 0 0 1 1 1
  spline S185 degree 2 poles (-31.2799, -62.1623) (-31.2799, -62.0383) (-31.1133, -62.0383) knots 0 0 0 1 1 1
  line L96 (-31.1133, -62.0383) -> (-30.1241, -62.0383)
  line L97 (-30.1241, -62.0383) -> (-30.1241, -58.7897)
  line L98 (-30.1241, -58.7897) -> (-30.8489, -58.7897)
  spline S186 degree 2 poles (-30.8489, -58.7897) (-31.0187, -58.7897) (-31.0187, -58.6623) knots 0 0 0 1 1 1
  spline S187 degree 2 poles (-31.0187, -58.6623) (-31.0187, -58.535) (-30.8489, -58.535) knots 0 0 0 1 1 1
  line L99 (-30.8489, -58.535) -> (-29.8727, -58.535)
  line L100 (-29.8727, -58.535) -> (-29.8727, -62.0383)
  line L101 (-29.8727, -62.0383) -> (-28.8867, -62.0383)
  spline S188 degree 2 poles (-28.8867, -62.0383) (-28.7169, -62.0383) (-28.7169, -62.1623) knots 0 0 0 1 1 1
  spline S189 degree 2 poles (-24.8414, -62.1623) (-24.8414, -62.2897) (-25.0112, -62.2897) knots 0 0 0 1 1 1
  line L102 (-25.0112, -62.2897) -> (-25.6021, -62.2897)
  line L103 (-25.6021, -62.2897) -> (-25.6021, -61.9272)
  spline S190 degree 2 poles (-25.6021, -61.9272) (-26.1507, -62.3876) (-26.771, -62.3876) knots 0 0 0 1 1 1
  spline S191 degree 2 poles (-26.771, -62.3876) (-27.166, -62.3876) (-27.4305, -62.195) knots 0 0 0 1 1 1
  spline S192 degree 2 poles (-27.4305, -62.195) (-27.7309, -61.9795) (-27.7309, -61.5975) knots 0 0 0 1 1 1
  spline S193 degree 2 poles (-27.7309, -61.5975) (-27.7309, -61.1339) (-27.2836, -60.8857) knots 0 0 0 1 1 1
  spline S194 degree 2 poles (-27.2836, -60.8857) (-26.9212, -60.6898) (-26.4184, -60.6898) knots 0 0 0 1 1 1
  spline S195 degree 2 poles (-26.4184, -60.6898) (-26.0592, -60.6898) (-25.6021, -60.7813) knots 0 0 0 1 1 1
  line L104 (-25.6021, -60.7813) -> (-25.6021, -60.3764)
  spline S196 degree 2 poles (-25.6021, -60.3764) (-25.6021, -60.1087) (-25.8666, -59.9716) knots 0 0 0 1 1 1
  spline S197 degree 2 poles (-25.8666, -59.9716) (-26.0756, -59.8638) (-26.3661, -59.8638) knots 0 0 0 1 1 1
  spline S198 degree 2 poles (-26.3661, -59.8638) (-26.6567, -59.8638) (-27.1889, -60.0336) knots 0 0 0 1 1 1
  spline S199 degree 2 poles (-27.1889, -60.0336) (-27.2803, -60.063) (-27.3097, -60.063) knots 0 0 0 1 1 1
  spline S200 degree 2 poles (-27.3097, -60.063) (-27.4272, -60.063) (-27.4272, -59.9389) knots 0 0 0 1 1 1
  spline S201 degree 2 poles (-27.4272, -59.9389) (-27.4272, -59.8867) (-27.3979, -59.8573) knots 0 0 0 1 1 1
  spline S202 degree 2 poles (-27.3979, -59.8573) (-27.3554, -59.8116) (-27.0583, -59.7332) knots 0 0 0 1 1 1
  spline S203 degree 2 poles (-27.0583, -59.7332) (-26.5882, -59.6091) (-26.3531, -59.6091) knots 0 0 0 1 1 1
  spline S204 degree 2 poles (-26.3531, -59.6091) (-25.9678, -59.6091) (-25.6805, -59.7953) knots 0 0 0 1 1 1
  spline S205 degree 2 poles (-25.6805, -59.7953) (-25.3475, -60.0075) (-25.3475, -60.3764) knots 0 0 0 1 1 1
  line L105 (-25.3475, -60.3764) -> (-25.3475, -62.0383)
  line L106 (-25.3475, -62.0383) -> (-25.0112, -62.0383)
  spline S206 degree 2 poles (-25.0112, -62.0383) (-24.8414, -62.0383) (-24.8414, -62.1623) knots 0 0 0 1 1 1
  line L107 (-25.6021, -61.591) -> (-25.6021, -61.0392)
  spline S207 degree 2 poles (-25.6021, -61.0392) (-25.945, -60.9412) (-26.3923, -60.9412) knots 0 0 0 1 1 1
  spline S208 degree 2 poles (-26.3923, -60.9412) (-26.9342, -60.9412) (-27.2477, -61.1763) knots 0 0 0 1 1 1
  spline S209 degree 2 poles (-27.2477, -61.1763) (-27.4795, -61.3526) (-27.4795, -61.5975) knots 0 0 0 1 1 1
  spline S210 degree 2 poles (-27.4795, -61.5975) (-27.4795, -61.8717) (-27.2575, -62.0121) knots 0 0 0 1 1 1
  spline S211 degree 2 poles (-27.2575, -62.0121) (-27.0714, -62.1362) (-26.784, -62.1362) knots 0 0 0 1 1 1
  spline S212 degree 2 poles (-26.784, -62.1362) (-26.1702, -62.1362) (-25.6021, -61.591) knots 0 0 0 1 1 1
  spline S213 degree 2 poles (-21.1651, -62.1623) (-21.1651, -62.2897) (-21.3316, -62.2897) knots 0 0 0 1 1 1
  line L108 (-21.3316, -62.2897) -> (-22.0042, -62.2897)
  spline S214 degree 2 poles (-22.0042, -62.2897) (-22.174, -62.2897) (-22.174, -62.1623) knots 0 0 0 1 1 1
  spline S215 degree 2 poles (-22.174, -62.1623) (-22.174, -62.0383) (-22.0042, -62.0383) knots 0 0 0 1 1 1
  line L109 (-22.0042, -62.0383) -> (-21.7952, -62.0383)
  line L110 (-21.7952, -62.0383) -> (-21.7952, -60.4972)
  spline S216 degree 2 poles (-21.7952, -60.4972) (-21.7952, -60.2034) (-22.0107, -60.0271) knots 0 0 0 1 1 1
  spline S217 degree 2 poles (-22.0107, -60.0271) (-22.2099, -59.8638) (-22.5103, -59.8638) knots 0 0 0 1 1 1
  spline S218 degree 2 poles (-22.5103, -59.8638) (-22.8139, -59.8638) (-23.0522, -60.0401) knots 0 0 0 1 1 1
  spline S219 degree 2 poles (-23.0522, -60.0401) (-23.1894, -60.1413) (-23.4604, -60.4613) knots 0 0 0 1 1 1
  line L111 (-23.4604, -60.4613) -> (-23.4604, -62.0383)
  line L112 (-23.4604, -62.0383) -> (-23.1763, -62.0383)
  spline S220 degree 2 poles (-23.1763, -62.0383) (-23.0098, -62.0383) (-23.0098, -62.1623) knots 0 0 0 1 1 1
  spline S221 degree 2 poles (-23.0098, -62.1623) (-23.0098, -62.2897) (-23.1763, -62.2897) knots 0 0 0 1 1 1
  line L113 (-23.1763, -62.2897) -> (-23.9958, -62.2897)
  spline S222 degree 2 poles (-23.9958, -62.2897) (-24.1623, -62.2897) (-24.1623, -62.1623) knots 0 0 0 1 1 1
  spline S223 degree 2 poles (-24.1623, -62.1623) (-24.1623, -62.0383) (-23.9958, -62.0383) knots 0 0 0 1 1 1
  line L114 (-23.9958, -62.0383) -> (-23.7118, -62.0383)
  line L115 (-23.7118, -62.0383) -> (-23.7118, -59.9552)
  line L116 (-23.7118, -59.9552) -> (-23.924, -59.9552)
  spline S224 degree 2 poles (-23.924, -59.9552) (-24.0905, -59.9552) (-24.0905, -59.8279) knots 0 0 0 1 1 1
  spline S225 degree 2 poles (-24.0905, -59.8279) (-24.0905, -59.7006) (-23.924, -59.7006) knots 0 0 0 1 1 1
  line L117 (-23.924, -59.7006) -> (-23.4604, -59.7006)
  line L118 (-23.4604, -59.7006) -> (-23.4604, -60.0793)
  spline S226 degree 2 poles (-23.4604, -60.0793) (-22.9967, -59.6091) (-22.507, -59.6091) knots 0 0 0 1 1 1
  spline S227 degree 2 poles (-22.507, -59.6091) (-21.952, -59.6091) (-21.6777, -60.0271) knots 0 0 0 1 1 1
  spline S228 degree 2 poles (-21.6777, -60.0271) (-21.5438, -60.236) (-21.5438, -60.4548) knots 0 0 0 1 1 1
  line L119 (-21.5438, -60.4548) -> (-21.5438, -62.0383)
  line L120 (-21.5438, -62.0383) -> (-21.3316, -62.0383)
  spline S229 degree 2 poles (-21.3316, -62.0383) (-21.1651, -62.0383) (-21.1651, -62.1623) knots 0 0 0 1 1 1
  spline S230 degree 2 poles (-17.6814, -62.1623) (-17.6814, -62.2897) (-17.8512, -62.2897) knots 0 0 0 1 1 1
  line L121 (-17.8512, -62.2897) -> (-20.0779, -62.2897)
  spline S231 degree 2 poles (-20.0779, -62.2897) (-20.2444, -62.2897) (-20.2444, -62.1623) knots 0 0 0 1 1 1
  spline S232 degree 2 poles (-20.2444, -62.1623) (-20.2444, -62.0383) (-20.0779, -62.0383) knots 0 0 0 1 1 1
  line L122 (-20.0779, -62.0383) -> (-19.0886, -62.0383)
  line L123 (-19.0886, -62.0383) -> (-19.0886, -59.9552)
  line L124 (-19.0886, -59.9552) -> (-19.8232, -59.9552)
  spline S233 degree 2 poles (-19.8232, -59.9552) (-19.993, -59.9552) (-19.993, -59.8279) knots 0 0 0 1 1 1
  spline S234 degree 2 poles (-19.993, -59.8279) (-19.993, -59.7006) (-19.8232, -59.7006) knots 0 0 0 1 1 1
  line L125 (-19.8232, -59.7006) -> (-18.8372, -59.7006)
  line L126 (-18.8372, -59.7006) -> (-18.8372, -62.0383)
  line L127 (-18.8372, -62.0383) -> (-17.8512, -62.0383)
  spline S235 degree 2 poles (-17.8512, -62.0383) (-17.6814, -62.0383) (-17.6814, -62.1623) knots 0 0 0 1 1 1
  line L128 (-18.8438, -59.0606) -> (-19.216, -59.0606)
  line L129 (-19.216, -59.0606) -> (-19.216, -58.4109)
  line L130 (-19.216, -58.4109) -> (-18.8438, -58.4109)
  line L131 (-18.8438, -58.4109) -> (-18.8438, -59.0606)
  spline S236 degree 2 poles (-13.8125, -62.1623) (-13.8125, -62.2897) (-13.979, -62.2897) knots 0 0 0 1 1 1
  line L132 (-13.979, -62.2897) -> (-14.6516, -62.2897)
  spline S237 degree 2 poles (-14.6516, -62.2897) (-14.8214, -62.2897) (-14.8214, -62.1623) knots 0 0 0 1 1 1
  spline S238 degree 2 poles (-14.8214, -62.1623) (-14.8214, -62.0383) (-14.6516, -62.0383) knots 0 0 0 1 1 1
  line L133 (-14.6516, -62.0383) -> (-14.4426, -62.0383)
  line L134 (-14.4426, -62.0383) -> (-14.4426, -60.4972)
  spline S239 degree 2 poles (-14.4426, -60.4972) (-14.4426, -60.2034) (-14.6581, -60.0271) knots 0 0 0 1 1 1
  spline S240 degree 2 poles (-14.6581, -60.0271) (-14.8573, -59.8638) (-15.1577, -59.8638) knots 0 0 0 1 1 1
  spline S241 degree 2 poles (-15.1577, -59.8638) (-15.4613, -59.8638) (-15.6996, -60.0401) knots 0 0 0 1 1 1
  spline S242 degree 2 poles (-15.6996, -60.0401) (-15.8368, -60.1413) (-16.1077, -60.4613) knots 0 0 0 1 1 1
  line L135 (-16.1077, -60.4613) -> (-16.1077, -62.0383)
  line L136 (-16.1077, -62.0383) -> (-15.8237, -62.0383)
  spline S243 degree 2 poles (-15.8237, -62.0383) (-15.6572, -62.0383) (-15.6572, -62.1623) knots 0 0 0 1 1 1
  spline S244 degree 2 poles (-15.6572, -62.1623) (-15.6572, -62.2897) (-15.8237, -62.2897) knots 0 0 0 1 1 1
  line L137 (-15.8237, -62.2897) -> (-16.6432, -62.2897)
  spline S245 degree 2 poles (-16.6432, -62.2897) (-16.8097, -62.2897) (-16.8097, -62.1623) knots 0 0 0 1 1 1
  spline S246 degree 2 poles (-16.8097, -62.1623) (-16.8097, -62.0383) (-16.6432, -62.0383) knots 0 0 0 1 1 1
  line L138 (-16.6432, -62.0383) -> (-16.3591, -62.0383)
  line L139 (-16.3591, -62.0383) -> (-16.3591, -59.9552)
  line L140 (-16.3591, -59.9552) -> (-16.5714, -59.9552)
  spline S247 degree 2 poles (-16.5714, -59.9552) (-16.7379, -59.9552) (-16.7379, -59.8279) knots 0 0 0 1 1 1
  spline S248 degree 2 poles (-16.7379, -59.8279) (-16.7379, -59.7006) (-16.5714, -59.7006) knots 0 0 0 1 1 1
  line L141 (-16.5714, -59.7006) -> (-16.1077, -59.7006)
  line L142 (-16.1077, -59.7006) -> (-16.1077, -60.0793)
  spline S249 degree 2 poles (-16.1077, -60.0793) (-15.6441, -59.6091) (-15.1544, -59.6091) knots 0 0 0 1 1 1
  spline S250 degree 2 poles (-15.1544, -59.6091) (-14.5993, -59.6091) (-14.3251, -60.0271) knots 0 0 0 1 1 1
  spline S251 degree 2 poles (-14.3251, -60.0271) (-14.1912, -60.236) (-14.1912, -60.4548) knots 0 0 0 1 1 1
  line L143 (-14.1912, -60.4548) -> (-14.1912, -62.0383)
  line L144 (-14.1912, -62.0383) -> (-13.979, -62.0383)
  spline S252 degree 2 poles (-13.979, -62.0383) (-13.8125, -62.0383) (-13.8125, -62.1623) knots 0 0 0 1 1 1
  spline S253 degree 2 poles (-10.1362, -62.1623) (-10.1362, -62.2897) (-10.306, -62.2897) knots 0 0 0 1 1 1
  line L145 (-10.306, -62.2897) -> (-10.8969, -62.2897)
  line L146 (-10.8969, -62.2897) -> (-10.8969, -61.9272)
  spline S254 degree 2 poles (-10.8969, -61.9272) (-11.4454, -62.3876) (-12.0658, -62.3876) knots 0 0 0 1 1 1
  spline S255 degree 2 poles (-12.0658, -62.3876) (-12.4608, -62.3876) (-12.7253, -62.195) knots 0 0 0 1 1 1
  spline S256 degree 2 poles (-12.7253, -62.195) (-13.0257, -61.9795) (-13.0257, -61.5975) knots 0 0 0 1 1 1
  spline S257 degree 2 poles (-13.0257, -61.5975) (-13.0257, -61.1339) (-12.5784, -60.8857) knots 0 0 0 1 1 1
  spline S258 degree 2 poles (-12.5784, -60.8857) (-12.216, -60.6898) (-11.7132, -60.6898) knots 0 0 0 1 1 1
  spline S259 degree 2 poles (-11.7132, -60.6898) (-11.354, -60.6898) (-10.8969, -60.7813) knots 0 0 0 1 1 1
  line L147 (-10.8969, -60.7813) -> (-10.8969, -60.3764)
  spline S260 degree 2 poles (-10.8969, -60.3764) (-10.8969, -60.1087) (-11.1614, -59.9716) knots 0 0 0 1 1 1
  spline S261 degree 2 poles (-11.1614, -59.9716) (-11.3703, -59.8638) (-11.6609, -59.8638) knots 0 0 0 1 1 1
  spline S262 degree 2 poles (-11.6609, -59.8638) (-11.9515, -59.8638) (-12.4837, -60.0336) knots 0 0 0 1 1 1
  spline S263 degree 2 poles (-12.4837, -60.0336) (-12.5751, -60.063) (-12.6045, -60.063) knots 0 0 0 1 1 1
  spline S264 degree 2 poles (-12.6045, -60.063) (-12.722, -60.063) (-12.722, -59.9389) knots 0 0 0 1 1 1
  spline S265 degree 2 poles (-12.722, -59.9389) (-12.722, -59.8867) (-12.6926, -59.8573) knots 0 0 0 1 1 1
  spline S266 degree 2 poles (-12.6926, -59.8573) (-12.6502, -59.8116) (-12.3531, -59.7332) knots 0 0 0 1 1 1
  spline S267 degree 2 poles (-12.3531, -59.7332) (-11.8829, -59.6091) (-11.6479, -59.6091) knots 0 0 0 1 1 1
  spline S268 degree 2 poles (-11.6479, -59.6091) (-11.2626, -59.6091) (-10.9753, -59.7953) knots 0 0 0 1 1 1
  spline S269 degree 2 poles (-10.9753, -59.7953) (-10.6423, -60.0075) (-10.6423, -60.3764) knots 0 0 0 1 1 1
  line L148 (-10.6423, -60.3764) -> (-10.6423, -62.0383)
  line L149 (-10.6423, -62.0383) -> (-10.306, -62.0383)
  spline S270 degree 2 poles (-10.306, -62.0383) (-10.1362, -62.0383) (-10.1362, -62.1623) knots 0 0 0 1 1 1
  line L150 (-10.8969, -61.591) -> (-10.8969, -61.0392)
  spline S271 degree 2 poles (-10.8969, -61.0392) (-11.2397, -60.9412) (-11.687, -60.9412) knots 0 0 0 1 1 1
  spline S272 degree 2 poles (-11.687, -60.9412) (-12.229, -60.9412) (-12.5424, -61.1763) knots 0 0 0 1 1 1
  spline S273 degree 2 poles (-12.5424, -61.1763) (-12.7743, -61.3526) (-12.7743, -61.5975) knots 0 0 0 1 1 1
  spline S274 degree 2 poles (-12.7743, -61.5975) (-12.7743, -61.8717) (-12.5522, -62.0121) knots 0 0 0 1 1 1
  spline S275 degree 2 poles (-12.5522, -62.0121) (-12.3661, -62.1362) (-12.0788, -62.1362) knots 0 0 0 1 1 1
  spline S276 degree 2 poles (-12.0788, -62.1362) (-11.465, -62.1362) (-10.8969, -61.591) knots 0 0 0 1 1 1
  dimension "d35" = 40
  dimension "d36" = 10
  dimension "d37" = 10
  dimension "d38" = 6
  constraints: 2 other
  measures "d35" distance of L2.start L2.end
  measures "d36" distance of L4.end L2.start
  measures "d37" distance between parallel lines of L1 L3
  measures "d38" distance between parallel lines of L0 L4
extrude "Extrusion6" cut sketch "Sketch6" against normal blind 0.001
equation "\"d22\" = d21"
body "Solid1"
